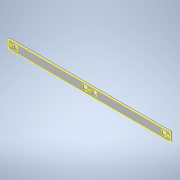
# Autodesk Inventor part: LED_Holder_FrontTop
Saved by Autodesk Inventor 2021 (Build 250183000, 183)
## iProperties
Created: 2021-02-24
Part Number: LED_Holder_FrontTop
Material: Generic
Document SubType Name: Modeling
Designer: Viktor
Density: 1 g/cm^3
Appearance: Default
Author: Viktor
Autodesk Inventor part; units mm, degrees
ref_plane "YZ Plane" through (0, 0, 0) normal (1, 0, 0) x (0, 1, 0)
ref_plane "XZ Plane" through (0, 0, 0) normal (0, 1, 0) x (-1, 0, 0)
ref_plane "XY Plane" through (0, 0, 0) normal (0, 0, 1) x (1, 0, 0)
sketch "Sketch1" plane through (0, 0, 0) normal (0, 0, 1) x (1, 0, 0)
  line L0 (-190, -10) -> (190, -10)
  line L1 (190, -10) -> (190, 10)
  line L2 (190, 10) -> (-190, 10)
  line L3 (-190, 10) -> (-190, -10)
  line L4 (-190, -10) -> (190, 10) construction
  line L5 (190, -10) -> (-190, 10) construction
  line L6 (-266.2899, 0) -> (266.2899, 0) construction
  line L7 (-178, -5.5) -> (-6, -5.5)
  line L8 (-6, -5.5) -> (-6, 5.5)
  line L9 (-6, 5.5) -> (-178, 5.5)
  line L10 (-178, 5.5) -> (-178, -5.5)
  line L11 (-178, -5.5) -> (-6, 5.5) construction
  line L12 (-6, -5.5) -> (-178, 5.5) construction
  line L13 (0, 14.2899) -> (0, -14.2899) construction
  line L14 (178, -5.5) -> (6, -5.5)
  line L15 (6, -5.5) -> (6, 5.5)
  line L16 (6, 5.5) -> (178, 5.5)
  line L17 (178, 5.5) -> (178, -5.5)
  line L18 (178, -5.5) -> (6, 5.5) construction
  line L19 (6, -5.5) -> (178, 5.5) construction
  circle A0 centre (-184, 0) radius 2.75
  circle A1 centre (0, 0) radius 2.75
  circle A2 centre (184, 0) radius 2.75
  line L20 (-178, 5.5) -> (-168, 5.5)
  line L21 (-168, 5.5) -> (-168, -5.5)
  line L22 (-168, -5.5) -> (-178, -5.5)
  line L23 (-178, -5.5) -> (-178, 5.5)
  line L24 (-6, 5.5) -> (-16, 5.5)
  line L25 (-16, 5.5) -> (-16, -5.5)
  line L26 (-16, -5.5) -> (-6, -5.5)
  line L27 (-6, -5.5) -> (-6, 5.5)
  line L28 (16, 5.5) -> (16, -5.5)
  line L29 (168, 5.5) -> (168, -5.5)
  point P0 (-92, 0)
  point P1 (92, 0)
  point P2 (168, -5.5)
  dimension "d0" = 380
  dimension "d1" = 20
  dimension "d2" = 11
  dimension "d3" = 12
  dimension "d4" = 6
  dimension "d5" = 5.5
  dimension "d6" = 6
  dimension "d7" = 5.5
  dimension "d11" = 10
  dimension "d12" = 10
  constraints: 56 end point, 10 symmetric about line, 8 parallel, 6 midpoint, 4 horizontal, 4 perpendicular, 4 point on line, 3 centre point, 1 coincident, 1 other
  measures "d0" distance between parallel lines of L1 L3
  measures "d1" distance between parallel lines of L0 L2
  measures "d2" distance between parallel lines of L7 L9
  measures "d3" distance between parallel lines of L3 L10
  measures "d4" horizontal distance of point (0, 0) L8.end
  measures "d5" diameter of A0
  measures "d6" distance from line of L10 A0.centre
  measures "d7" diameter of A1
  measures "d11" distance between parallel lines of L10 L21
  measures "d12" distance between parallel lines of L8 L25
extrude "Extrusion1" add sketch "Sketch1" along normal blind 3 contours L3 L2 L1 L0 | L21 L9 L25 L7 | L14 L28 L16 L29
fillet "Fillet1" radius 1 4 edges at (-190, -10, 1.5) (-190, 10, 1.5) (190, -10, 1.5) (190, 10, 1.5)
sketch "Sketch2" plane through (0, 0, 3) normal (0, 0, 1) x (1, 0, 0)
  arc A0 (190, 9) -> (189, 10) centre (189, 9) ccw projected
  line L0 (189, 10) -> (-189, 10) projected
  arc A1 (-189, 10) -> (-190, 9) centre (-189, 9) ccw projected
  line L1 (-190, 9) -> (-190, -9) projected
  arc A2 (-190, -9) -> (-189, -10) centre (-189, -9) ccw projected
  line L2 (-189, -10) -> (189, -10) projected
  arc A3 (189, -10) -> (190, -9) centre (189, -9) ccw projected
  line L3 (190, -9) -> (190, 9) projected
  circle A4 centre (-184, 0) radius 2.75 projected
  circle A5 centre (0, 0) radius 2.75 projected
  circle A6 centre (184, 0) radius 2.75 projected
  line L4 (16, 5.5) -> (16, -5.5) projected
  line L5 (16, -5.5) -> (6, -5.5) projected
  line L6 (6, -5.5) -> (6, 5.5) projected
  line L7 (6, 5.5) -> (16, 5.5) projected
  line L8 (-168, 5.5) -> (-168, -5.5) projected
  line L9 (-168, -5.5) -> (-178, -5.5) projected
  line L10 (-178, -5.5) -> (-178, 5.5) projected
  line L11 (-178, 5.5) -> (-168, 5.5) projected
  line L12 (168, 5.5) -> (178, 5.5) projected
  line L13 (178, 5.5) -> (178, -5.5) projected
  line L14 (178, -5.5) -> (168, -5.5) projected
  line L15 (168, -5.5) -> (168, 5.5) projected
  line L16 (-16, 5.5) -> (-6, 5.5) projected
  line L17 (-6, 5.5) -> (-6, -5.5) projected
  line L18 (-6, -5.5) -> (-16, -5.5) projected
  line L19 (-16, -5.5) -> (-16, 5.5) projected
equation "\"d6\" = 0.5 * d3"
equation "\"d7\" = d5"
equation "\"d12\" = d11"
body "Solid1"
